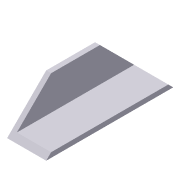
# Autodesk Inventor part: FE-00014-05
Saved by Autodesk Inventor 2012 (Build 160160000, 160)
## iProperties
Company: FIRST
Created: 2008-05-25
Part Number: FE-00014-05
Document SubType Name: Modeling
Designer: dfoster
Density: 1 g/cm^3
Description: Gusset
Mass: 10.2099 g
Surface Area: 72.2203 cm^2
Volume: 10.2099 cm^3
Material: Default
Title: Gusset
Author: dfoster
Autodesk Inventor part; units mm, degrees
ref_plane "YZ Plane" through (0, 0, 0) normal (1, 0, 0) x (0, 1, 0)
ref_plane "XZ Plane" through (0, 0, 0) normal (0, 1, 0) x (-1, 0, 0)
ref_plane "XY Plane" through (0, 0, 0) normal (0, 0, 1) x (1, 0, 0)
sketch "Sketch1" plane through (0, 0, 0) normal (0, 0, 1) x (1, 0, 0)
  line L0 (-26.7607, 27.2143) -> (-26.7607, 1.8143)
  line L1 (-26.7607, 1.8143) -> (-1.3607, 1.8143)
  line L2 (-1.3607, 1.8143) -> (-1.3607, 4.9893)
  line L3 (-1.3607, 4.9893) -> (-23.5857, 4.9893)
  line L4 (-23.5857, 4.9893) -> (-23.5857, 27.2143)
  line L5 (-23.5857, 27.2143) -> (-26.7607, 27.2143)
  dimension "d0" = 25.4
  dimension "d1" = 3.175
  constraints: 12 end point, 4 parallel, 3 perpendicular, 1 vertical
  measures "d0" distance of L0.start L0.end
  measures "d1" distance of L4.end L0.start
extrude "Extrusion1" add sketch "Sketch1" along normal blind 82.55
chamfer "Chamfer1" distance 25.4 angle 45 2 edges at (-25.1732, 27.2143, 82.55) (-25.1732, 27.2143, 0)
body "Solid1"
